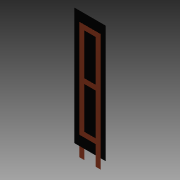
# Autodesk Inventor part: Captor
Saved by Autodesk Inventor 2014 SP1 (Build 180222100, 222)
## iProperties
Created: 2015-03-28
Part Number: Captor
Material: Generic
Document SubType Name: Modeling
Designer: tuleu
Density: 1 g/cm^3
Appearance: Default
Author: tuleu
Autodesk Inventor part; units mm, degrees
ref_plane "YZ Plane" through (0, 0, 0) normal (1, 0, 0) x (0, 1, 0)
ref_plane "XZ Plane" through (0, 0, 0) normal (0, 1, 0) x (-1, 0, 0)
ref_plane "XY Plane" through (0, 0, 0) normal (0, 0, 1) x (1, 0, 0)
sketch "Sketch1" plane through (0, 0, 0) normal (0, 1, 0) x (-1, 0, 0)
  line L0 (40, -150) -> (-40, -150)
  line L1 (-40, -150) -> (-40, 150)
  line L2 (-40, 150) -> (40, 150)
  line L3 (40, 150) -> (40, -150)
  line L4 (0, -150) -> (0, 150)
  line L5 (40, 0) -> (-40, 0)
  point P0 (0, 0)
  dimension "d0" = 300
  dimension "d1" = 80
  constraints: 12 end point, 6 midpoint, 3 perpendicular, 2 parallel, 1 horizontal, 2 other
  measures "d0" distance of L2.end L0.start
  measures "d1" distance of L0.start L0.end
extrude "Extrusion1" add sketch "Sketch1" along normal blind 0.1
sketch "Sketch2" plane through (0, 0.1, 0) normal (0, 1, 0) x (1, 0, 0)
  line L0 (-40, -150) -> (40, -150) projected
  line L1 (40, -150) -> (40, 150) projected
  line L2 (40, 150) -> (-40, 150) projected
  line L3 (-40, 150) -> (-40, -150) projected
  line L4 (-27.5, 175) -> (-27.5, -125)
  line L5 (-27.5, -125) -> (27.5, -125)
  line L6 (27.5, -125) -> (27.5, 125)
  line L7 (27.5, 125) -> (-14.8, 125)
  line L8 (-14.8, 125) -> (-14.8, 175)
  line L9 (-14.8, 175) -> (-27.5, 175)
  line L10 (-14.8, 112.3) -> (-14.8, 6.35)
  line L11 (-14.8, 6.35) -> (14.8, 6.35)
  line L12 (14.8, 6.35) -> (14.8, 112.3)
  line L13 (14.8, 112.3) -> (-14.8, 112.3)
  line L14 (-14.8, -6.35) -> (14.8, -6.35)
  line L15 (14.8, -6.35) -> (14.8, -112.3)
  line L16 (14.8, -112.3) -> (-14.8, -112.3)
  line L17 (-14.8, -112.3) -> (-14.8, -6.35)
  line L18 (-40, 0) -> (40, 0)
  point P0 (0, 0)
  dimension "d4" = 12.7
  dimension "d5" = 12.7
  dimension "d6" = 12.7
  dimension "d7" = 12.7
  dimension "d8" = 12.7
  dimension "d9" = 25
  dimension "d10" = 25
  dimension "d11" = 12.5
  dimension "d12" = 12.5
  dimension "d13" = 250
  dimension "d14" = 50
  constraints: 30 end point, 7 parallel, 7 perpendicular, 3 collinear, 2 midpoint, 1 other
  measures "d4" distance between parallel lines of L8 L4
  measures "d5" distance between parallel lines of L13 L7
  measures "d6" distance between parallel lines of L6 L12
  measures "d7" distance between parallel lines of L11 L14
  measures "d8" distance between parallel lines of L5 L16
  measures "d9" distance between parallel lines of L0 L5
  measures "d10" distance between parallel lines of L2 L7
  measures "d11" distance between parallel lines of L1 L6
  measures "d12" distance between parallel lines of L3 L4
  measures "d13" distance between parallel lines of L5 L7
  measures "d14" distance from line of L7 L4.start
extrude "Extrusion2" add sketch "Sketch2" along normal blind 0.1 contours L18 L6 L5 L4 | L4 L2 L8 L7 L6 L18 | L4 L9 L8 L2
sketch "Sketch3" plane through (0, 0, 0) normal (0, -1, 0) x (1, 0, 0)
  line L0 (40, -150) -> (-40, -150) projected
  line L1 (27.5, 125) -> (27.5, -175)
  line L2 (27.5, -175) -> (14.8, -175)
  line L3 (14.8, -175) -> (14.8, -125)
  line L4 (14.8, -125) -> (-27.5, -125)
  line L5 (-27.5, -125) -> (-27.5, 125)
  line L6 (-27.5, 125) -> (27.5, 125)
  line L7 (-14.8, 112.3) -> (14.8, 112.3)
  line L8 (14.8, 112.3) -> (14.8, 6.35)
  line L9 (14.8, 6.35) -> (-14.8, 6.35)
  line L10 (-14.8, 6.35) -> (-14.8, 112.3)
  line L11 (-14.8, -6.35) -> (14.8, -6.35)
  line L12 (14.8, -6.35) -> (14.8, -112.3)
  line L13 (14.8, -112.3) -> (-14.8, -112.3)
  line L14 (-14.8, -112.3) -> (-14.8, -6.35)
  line L15 (27.5, 125) -> (-27.5, 125) projected
  line L16 (-14.8, 112.3) -> (14.8, 112.3) projected
  line L17 (-27.5, 125) -> (-27.5, -150) projected
  line L18 (27.5, -125) -> (27.5, 125) projected
  line L19 (-14.8, -125) -> (27.5, -125) projected
  line L20 (14.8, -6.35) -> (14.8, -112.3) projected
  line L21 (-14.8, -112.3) -> (-14.8, -6.35) projected
  line L22 (-14.8, -6.35) -> (14.8, -6.35) projected
  line L23 (14.8, 6.35) -> (-14.8, 6.35) projected
  line L24 (14.8, -112.3) -> (-14.8, -112.3) projected
  line L25 (-14.8, -175) -> (-27.5, -175) projected
  point P0 (0, 0)
  constraints: 28 end point, 14 collinear, 8 parallel, 4 perpendicular, 2 horizontal
extrude "Extrusion3" add sketch "Sketch3" along normal blind 0.1 contours L1 L2 L3 L0 | L0 L3 L19 L1 | L19 L4 L5 L6 L1
body "Solid1"
